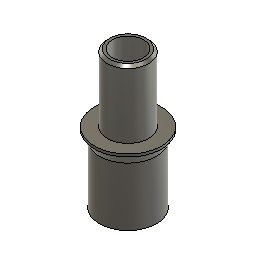
Alcohol Tester v4 (Autodesk Fusion 360 design; units mm, degrees)
Autodesk Fusion 360 part; units mm, degrees
sketch "Sketch1" plane through (0, 0, 0) normal (0, 0, 1) x (1, 0, 0)
  line L0 (4, 0) -> (4, 10.2679)
  line L1 (4, 10.2679) -> (3, 12)
  line L2 (1.5, 21.5) -> (3, 21.5)
  line L3 (3, 21.5) -> (3, 26.5)
  line L4 (3, 26.5) -> (4, 26.5)
  line L5 (4, 26.5) -> (4, 13.5)
  line L6 (4, 13.5) -> (6.5, 13.5)
  line L7 (6.5, 13.5) -> (6.5, 13)
  line L8 (6.5, 13) -> (5.5, 11.2679)
  line L9 (5.5, 11.2679) -> (5.5, 0)
  line L10 (5.5, 0) -> (4, 0)
  line L11 (0, 0) -> (0, 26.5) construction
  line L12 (3, 12) -> (3, 17.9019)
  line L13 (1.5, 21.5) -> (1.5, 20.5)
  line L14 (1.5, 20.5) -> (3, 17.9019)
  dimension "d2" = 4
  dimension "d3" = 5.5
  dimension "d4" = 3
  dimension "d5" = 4
  dimension "d6" = 6.5
  dimension "d7" = 13
  dimension "d9" = 12
  dimension "d10" = 5
  dimension "d11" = 13
  dimension "d12" = 26.5
  dimension "d13" = 60
  dimension "d14" = 60
  dimension "d15" = 3
  dimension "d16" = 1.5
  dimension "d17" = 60
  dimension "d18" = 6
  constraint vertical L0
  constraint perpendicular L2 L3
  constraint perpendicular L3 L4
  constraint perpendicular L4 L5
  constraint perpendicular L0 L6
  constraint perpendicular L6 L7
  constraint perpendicular L6 L9
  constraint perpendicular L0 L10
  constraint coincident L11.start origin
  constraint vertical L11
  constraint horizontal L11.start L0.start
  constraint horizontal L3.end L11.end
  constraint parallel L5 L12
  constraint perpendicular L2 L13
  measures "d2" distance of L0 L11
  measures "d3" distance of L9 L11
  measures "d4" distance of L3 L11
  measures "d5" distance of L5 L11
  measures "d6" distance of L7 L11
  measures "d7" vertical distance of L11.start L7.end
  measures "d9" vertical distance of L11.start L1.end
  measures "d10" distance of L2 L4
  measures "d11" distance of L4 L6
  measures "d12" distance of L4 L10
  measures "d13" angle of L1 L10
  measures "d14" angle of L6 L8
  measures "d15" distance of L11 L12
  measures "d16" distance of L11 L13
  measures "d17" angle of L2 L14
  measures "d18" distance of L4 L13.end
revolve "Revolve1" add sketch "Sketch1" angle 360 about axis through (0, 0, 0) along (0, 1, 0)
chamfer "Chamfer1" distance 0.5 angle 45 1 edges at (-3.7293, 26.5, -1.4465)
equation "d2 = ( 8 / 2 ) * 1 mm"
equation "d3 = ( 11 / 2 ) * 1 mm"
equation "d4 = ( 6 / 2 ) * 1 mm"
equation "d5 = ( 8 / 2 ) * 1 mm"
equation "d6 = ( 13 / 2 ) * 1 mm"
equation "d15 = ( 6 / 2 ) * 1 mm"
equation "d16 = ( 3 / 2 ) * 1 mm"
named bodies: "AlcoholTesterTube"
